Autodesk Inventor part; units mm, degrees
(part 2 of 2)
  line L91 (2.1197, 26) -> (0.7473, 26) construction
  ellipse E127 centre (2.1197, 24) end of major axis (2.1197, 26) minor radius 1.9997 (2.1197, 22) -> (2.1197, 26) ccw construction
  line L92 (0.7473, 22) -> (2.1197, 22) construction
  ellipse E128 centre (0.7473, 24) end of major axis (0.7473, 22) minor radius 1.9997 (0.7473, 26) -> (0.7473, 22) ccw construction
  line L93 (26.1163, 26) -> (24.7439, 26) construction
  ellipse E129 centre (26.1163, 24) end of major axis (26.1163, 26) minor radius 1.9997 (26.1163, 22) -> (26.1163, 26) ccw construction
  line L94 (24.7439, 22) -> (26.1163, 22) construction
  ellipse E130 centre (24.7439, 24) end of major axis (24.7439, 22) minor radius 1.9997 (24.7439, 26) -> (24.7439, 22) ccw construction
  line L95 (50.1128, 26) -> (48.7405, 26) construction
  ellipse E131 centre (50.1128, 24) end of major axis (50.1128, 26) minor radius 1.9997 (50.1128, 22) -> (50.1128, 26) ccw construction
  line L96 (48.7405, 22) -> (50.1128, 22) construction
  ellipse E132 centre (48.7405, 24) end of major axis (48.7405, 22) minor radius 1.9997 (48.7405, 26) -> (48.7405, 22) ccw construction
  line L97 (74.1094, 26) -> (72.737, 26) construction
  ellipse E133 centre (74.1094, 24) end of major axis (74.1094, 26) minor radius 1.9997 (74.1094, 22) -> (74.1094, 26) ccw construction
  line L98 (72.737, 22) -> (74.1094, 22) construction
  ellipse E134 centre (72.737, 24) end of major axis (72.737, 22) minor radius 1.9997 (72.737, 26) -> (72.737, 22) ccw construction
  line L99 (98.106, 26) -> (96.7336, 26) construction
  ellipse E135 centre (98.106, 24) end of major axis (98.106, 26) minor radius 1.9997 (98.106, 22) -> (98.106, 26) ccw construction
  line L100 (96.7336, 22) -> (98.106, 22) construction
  ellipse E136 centre (96.7336, 24) end of major axis (96.7336, 22) minor radius 1.9997 (96.7336, 26) -> (96.7336, 22) ccw construction
  line L101 (122.1025, 26) -> (120.7302, 26) construction
  ellipse E137 centre (122.1025, 24) end of major axis (122.1025, 26) minor radius 1.9997 (122.1025, 22) -> (122.1025, 26) ccw construction
  line L102 (120.7302, 22) -> (122.1025, 22) construction
  ellipse E138 centre (120.7302, 24) end of major axis (120.7302, 22) minor radius 1.9997 (120.7302, 26) -> (120.7302, 22) ccw construction
  line L103 (146.0991, 26) -> (144.7267, 26) construction
  ellipse E139 centre (146.0991, 24) end of major axis (146.0991, 26) minor radius 1.9997 (146.0991, 22) -> (146.0991, 26) ccw construction
  line L104 (144.7267, 22) -> (146.0991, 22) construction
  ellipse E140 centre (144.7267, 24) end of major axis (144.7267, 22) minor radius 1.9997 (144.7267, 26) -> (144.7267, 22) ccw construction
  line L105 (170.0957, 26) -> (168.7233, 26) construction
  ellipse E141 centre (170.0957, 24) end of major axis (170.0957, 26) minor radius 1.9997 (170.0957, 22) -> (170.0957, 26) ccw construction
  line L106 (168.7233, 22) -> (170.0957, 22) construction
  ellipse E142 centre (168.7233, 24) end of major axis (168.7233, 22) minor radius 1.9997 (168.7233, 26) -> (168.7233, 22) ccw construction
  ellipse E143 centre (-43.0454, 32.4853) end of major axis (-43.0454, 34.4853) minor radius 1.9997 (-41.6314, 33.8995) -> (-44.4594, 31.0711) ccw construction
  line L107 (-41.1462, 33.4142) -> (-41.6314, 33.8995) construction
  ellipse E144 centre (-42.5602, 32) end of major axis (-42.5602, 30) minor radius 1.9997 (-43.9742, 30.5858) -> (-41.1462, 33.4142) ccw construction
  line L108 (-44.4594, 31.0711) -> (-43.9742, 30.5858) construction
  ellipse E145 centre (-19.0488, 32.4853) end of major axis (-19.0488, 34.4853) minor radius 1.9997 (-17.6348, 33.8995) -> (-20.4628, 31.0711) ccw construction
  line L109 (-17.1496, 33.4142) -> (-17.6348, 33.8995) construction
  ellipse E146 centre (-18.5636, 32) end of major axis (-18.5636, 30) minor radius 1.9997 (-19.9776, 30.5858) -> (-17.1496, 33.4142) ccw construction
  line L110 (-20.4628, 31.0711) -> (-19.9776, 30.5858) construction
  ellipse E147 centre (4.9477, 32.4853) end of major axis (4.9477, 34.4853) minor radius 1.9997 (6.3617, 33.8995) -> (3.5337, 31.0711) ccw construction
  line L111 (6.847, 33.4142) -> (6.3617, 33.8995) construction
  ellipse E148 centre (5.4329, 32) end of major axis (5.4329, 30) minor radius 1.9997 (4.0189, 30.5858) -> (6.847, 33.4142) ccw construction
  line L112 (3.5337, 31.0711) -> (4.0189, 30.5858) construction
  ellipse E149 centre (28.9443, 32.4853) end of major axis (28.9443, 34.4853) minor radius 1.9997 (30.3583, 33.8995) -> (27.5303, 31.0711) ccw construction
  line L113 (30.8435, 33.4142) -> (30.3583, 33.8995) construction
  ellipse E150 centre (29.4295, 32) end of major axis (29.4295, 30) minor radius 1.9997 (28.0155, 30.5858) -> (30.8435, 33.4142) ccw construction
  line L114 (27.5303, 31.0711) -> (28.0155, 30.5858) construction
  ellipse E151 centre (52.9409, 32.4853) end of major axis (52.9409, 34.4853) minor radius 1.9997 (54.3549, 33.8995) -> (51.5269, 31.0711) ccw construction
  line L115 (54.8401, 33.4142) -> (54.3549, 33.8995) construction
  ellipse E152 centre (53.4261, 32) end of major axis (53.4261, 30) minor radius 1.9997 (52.0121, 30.5858) -> (54.8401, 33.4142) ccw construction
  line L116 (51.5269, 31.0711) -> (52.0121, 30.5858) construction
  ellipse E153 centre (76.9374, 32.4853) end of major axis (76.9374, 34.4853) minor radius 1.9997 (78.3514, 33.8995) -> (75.5234, 31.0711) ccw construction
  line L117 (78.8367, 33.4142) -> (78.3514, 33.8995) construction
  ellipse E154 centre (77.4226, 32) end of major axis (77.4226, 30) minor radius 1.9997 (76.0086, 30.5858) -> (78.8367, 33.4142) ccw construction
  line L118 (75.5234, 31.0711) -> (76.0086, 30.5858) construction
  ellipse E155 centre (100.934, 32.4853) end of major axis (100.934, 34.4853) minor radius 1.9997 (102.348, 33.8995) -> (99.52, 31.0711) ccw construction
  line L119 (102.8332, 33.4142) -> (102.348, 33.8995) construction
  ellipse E156 centre (101.4192, 32) end of major axis (101.4192, 30) minor radius 1.9997 (100.0052, 30.5858) -> (102.8332, 33.4142) ccw construction
  line L120 (99.52, 31.0711) -> (100.0052, 30.5858) construction
  ellipse E157 centre (124.9306, 32.4853) end of major axis (124.9306, 34.4853) minor radius 1.9997 (126.3446, 33.8995) -> (123.5166, 31.0711) ccw construction
  line L121 (126.8298, 33.4142) -> (126.3446, 33.8995) construction
  ellipse E158 centre (125.4158, 32) end of major axis (125.4158, 30) minor radius 1.9997 (124.0018, 30.5858) -> (126.8298, 33.4142) ccw construction
  line L122 (123.5166, 31.0711) -> (124.0018, 30.5858) construction
  ellipse E159 centre (148.9271, 32.4853) end of major axis (148.9271, 34.4853) minor radius 1.9997 (150.3411, 33.8995) -> (147.5131, 31.0711) ccw construction
  line L123 (150.8264, 33.4142) -> (150.3411, 33.8995) construction
  ellipse E160 centre (149.4123, 32) end of major axis (149.4123, 30) minor radius 1.9997 (147.9983, 30.5858) -> (150.8264, 33.4142) ccw construction
  line L124 (147.5131, 31.0711) -> (147.9983, 30.5858) construction
  ellipse E161 centre (172.9237, 32.4853) end of major axis (172.9237, 34.4853) minor radius 1.9997 (174.3377, 33.8995) -> (171.5097, 31.0711) ccw construction
  line L125 (174.8229, 33.4142) -> (174.3377, 33.8995) construction
  ellipse E162 centre (173.4089, 32) end of major axis (173.4089, 30) minor radius 1.9997 (171.9949, 30.5858) -> (174.8229, 33.4142) ccw construction
  line L126 (171.5097, 31.0711) -> (171.9949, 30.5858) construction
  ellipse E163 centre (-26.0773, 15.5147) end of major axis (-26.0773, 17.5147) minor radius 1.9997 (-27.4913, 14.1005) -> (-24.6632, 16.9289) ccw construction
  line L127 (-27.9765, 14.5858) -> (-27.4913, 14.1005) construction
  ellipse E164 centre (-26.5625, 16) end of major axis (-26.5625, 18) minor radius 1.9997 (-25.1485, 17.4142) -> (-27.9765, 14.5858) ccw construction
  line L128 (-24.6632, 16.9289) -> (-25.1485, 17.4142) construction
  ellipse E165 centre (-2.0807, 15.5147) end of major axis (-2.0807, 17.5147) minor radius 1.9997 (-3.4947, 14.1005) -> (-0.6667, 16.9289) ccw construction
  line L129 (-3.9799, 14.5858) -> (-3.4947, 14.1005) construction
  ellipse E166 centre (-2.5659, 16) end of major axis (-2.5659, 18) minor radius 1.9997 (-1.1519, 17.4142) -> (-3.9799, 14.5858) ccw construction
  line L130 (-0.6667, 16.9289) -> (-1.1519, 17.4142) construction
  ellipse E167 centre (21.9159, 15.5147) end of major axis (21.9159, 17.5147) minor radius 1.9997 (20.5019, 14.1005) -> (23.3299, 16.9289) ccw construction
  line L131 (20.0166, 14.5858) -> (20.5019, 14.1005) construction
  ellipse E168 centre (21.4307, 16) end of major axis (21.4307, 18) minor radius 1.9997 (22.8447, 17.4142) -> (20.0166, 14.5858) ccw construction
  line L132 (23.3299, 16.9289) -> (22.8447, 17.4142) construction
  ellipse E169 centre (45.9124, 15.5147) end of major axis (45.9124, 17.5147) minor radius 1.9997 (44.4984, 14.1005) -> (47.3264, 16.9289) ccw construction
  line L133 (44.0132, 14.5858) -> (44.4984, 14.1005) construction
  ellipse E170 centre (45.4272, 16) end of major axis (45.4272, 18) minor radius 1.9997 (46.8412, 17.4142) -> (44.0132, 14.5858) ccw construction
  line L134 (47.3264, 16.9289) -> (46.8412, 17.4142) construction
  ellipse E171 centre (69.909, 15.5147) end of major axis (69.909, 17.5147) minor radius 1.9997 (68.495, 14.1005) -> (71.323, 16.9289) ccw construction
  line L135 (68.0098, 14.5858) -> (68.495, 14.1005) construction
  ellipse E172 centre (69.4238, 16) end of major axis (69.4238, 18) minor radius 1.9997 (70.8378, 17.4142) -> (68.0098, 14.5858) ccw construction
  line L136 (71.323, 16.9289) -> (70.8378, 17.4142) construction
  ellipse E173 centre (93.9056, 15.5147) end of major axis (93.9056, 17.5147) minor radius 1.9997 (92.4916, 14.1005) -> (95.3196, 16.9289) ccw construction
  line L137 (92.0063, 14.5858) -> (92.4916, 14.1005) construction
  ellipse E174 centre (93.4204, 16) end of major axis (93.4204, 18) minor radius 1.9997 (94.8344, 17.4142) -> (92.0063, 14.5858) ccw construction
  line L138 (95.3196, 16.9289) -> (94.8344, 17.4142) construction
  ellipse E175 centre (117.9021, 15.5147) end of major axis (117.9021, 17.5147) minor radius 1.9997 (116.4881, 14.1005) -> (119.3161, 16.9289) ccw construction
  line L139 (116.0029, 14.5858) -> (116.4881, 14.1005) construction
  ellipse E176 centre (117.4169, 16) end of major axis (117.4169, 18) minor radius 1.9997 (118.8309, 17.4142) -> (116.0029, 14.5858) ccw construction
  line L140 (119.3161, 16.9289) -> (118.8309, 17.4142) construction
  ellipse E177 centre (141.8987, 15.5147) end of major axis (141.8987, 17.5147) minor radius 1.9997 (140.4847, 14.1005) -> (143.3127, 16.9289) ccw construction
  line L141 (139.9995, 14.5858) -> (140.4847, 14.1005) construction
  ellipse E178 centre (141.4135, 16) end of major axis (141.4135, 18) minor radius 1.9997 (142.8275, 17.4142) -> (139.9995, 14.5858) ccw construction
  line L142 (143.3127, 16.9289) -> (142.8275, 17.4142) construction
  ellipse E179 centre (165.8953, 15.5147) end of major axis (165.8953, 17.5147) minor radius 1.9997 (164.4813, 14.1005) -> (167.3093, 16.9289) ccw construction
  line L143 (163.996, 14.5858) -> (164.4813, 14.1005) construction
  ellipse E180 centre (165.4101, 16) end of major axis (165.4101, 18) minor radius 1.9997 (166.8241, 17.4142) -> (163.996, 14.5858) ccw construction
  line L144 (167.3093, 16.9289) -> (166.8241, 17.4142) construction
  ellipse E181 centre (-34.5613, 24) end of major axis (-34.5613, 31) minor radius 6.999 construction
  ellipse E182 centre (-10.5648, 24) end of major axis (-10.5648, 31) minor radius 6.999 construction
  ellipse E183 centre (13.4318, 24) end of major axis (13.4318, 31) minor radius 6.999 construction
  ellipse E184 centre (37.4284, 24) end of major axis (37.4284, 31) minor radius 6.999 construction
  ellipse E185 centre (61.4249, 24) end of major axis (61.4249, 31) minor radius 6.999 construction
  ellipse E186 centre (85.4215, 24) end of major axis (85.4215, 31) minor radius 6.999 construction
  ellipse E187 centre (109.4181, 24) end of major axis (109.4181, 31) minor radius 6.999 construction
  ellipse E188 centre (133.4146, 24) end of major axis (133.4146, 31) minor radius 6.999 construction
  ellipse E189 centre (157.4112, 24) end of major axis (157.4112, 31) minor radius 6.999 construction
  circle A0 centre (181.4078, 8) radius 2.2
  circle A1 centre (157.4112, 8) radius 2.2
  line L145 (181.525, 0) -> (181.525, 40.825) projected
  circle A2 centre (181.525, 36.5125) radius 2.2
  circle A3 centre (157.4112, 37.6569) radius 2.2
  point P0 (0, 0)
  dimension "d18" = 4.4
  dimension "d19" = 4.4
  dimension "d20" = 4.4
  dimension "d21" = 4.4
  constraints: 4 centre point, 2 coincident, 1 point on line, 141 other
  measures "d18" diameter of A0
  measures "d19" diameter of A1
  measures "d20" diameter of A2
  measures "d21" diameter of A3
extrude "Extrusion4" cut sketch "Sketch5" against normal through all
body "Solid1"
